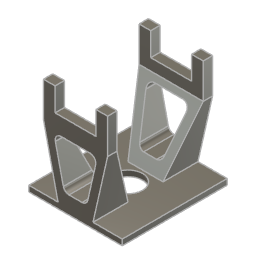
Jacks Stands F (Autodesk Fusion 360 design; units mm, degrees)
Autodesk Fusion 360 part; units mm, degrees
note: some values were not read from the file. Set by a fixed rule: which sketch regions a step uses.
sketch "Esquisse1" plane through (0, 0, 0) normal (0, 0, 1) x (1, 0, 0)
  line L0 (22.5, 70) -> (57.5, 70)
  line L1 (57.5, 70) -> (57.5, 90)
  line L2 (22.5, 70) -> (22.5, 90)
  line L3 (22.5, 90) -> (12.5, 90)
  line L4 (57.5, 90) -> (67.5, 90)
  line L5 (67.5, 90) -> (67.5, 60)
  line L6 (12.5, 90) -> (12.5, 60)
  line L7 (12.5, 60) -> (25, 5)
  line L8 (25, 5) -> (0, 5)
  line L9 (0, 5) -> (0, 0)
  line L10 (0, 0) -> (80, 0)
  line L11 (80, 0) -> (80, 5)
  line L12 (80, 5) -> (55, 5)
  line L13 (55, 5) -> (67.5, 60)
  dimension "d1" = 70
  dimension "d2" = 35
  dimension "d3" = 20
  dimension "d4" = 10
  dimension "d5" = 30
  dimension "d8" = 5
  dimension "d10" = 10
  dimension "d27" = 80
  dimension "d28" = 55
  dimension "d29" = 12.5
  dimension "d30" = 30
  constraint horizontal L0
  constraint perpendicular L0 L1
  constraint perpendicular L0 L2
  constraint perpendicular L2 L3
  constraint perpendicular L1 L4
  constraint perpendicular L4 L5
  constraint equal L3 L4
  constraint perpendicular L3 L6
  constraint perpendicular L6 L8
  constraint coincident L9.end L10.start
  constraint perpendicular L8 L9
  constraint perpendicular L9 L10
  constraint perpendicular L10 L11
  constraint perpendicular L9 L12
  constraint horizontal L5.end L6.end
  constraint equal L8 L12
  constraint collinear L8 L12
  measures "d1" distance of L9.end L0
  measures "d2" distance of L0.start L0.end
  measures "d3" distance of L0.end L1.end
  measures "d4" distance of L2.end L3.end
  measures "d5" distance of L3.end L6.end
  measures "d8" distance of L8 L10
  measures "d10" vertical distance of L0.end L5.end
  measures "d27" distance of L9.end L10.end
  measures "d28" distance of L5 L6
  measures "d29" distance of L5 L11
  measures "d30" distance of L7.end L12.end
extrude "Extrusion1" add sketch "Esquisse1" along normal blind 90
sketch "Esquisse2" plane through (67.5, 0, 0) normal (1, 0, 0) x (0, 0, -1)
  line L0 (0, 60) -> (0, 90)
  line L1 (0, 90) -> (-90, 90)
  line L2 (-90, 90) -> (-90, 60)
  line L3 (-90, 60) -> (0, 60)
  line L4 (-45, 90) -> (-45, -26) construction
  line L5 (-82, 90) -> (-82, 60)
  line L6 (-82, 60) -> (-60, 5)
  line L7 (-8, 90) -> (-8, 60)
  line L8 (-8, 60) -> (-30, 5)
  line L9 (-60, 5) -> (-30, 5)
  point P0 (-90, 5)
  point P1 (0, 5)
  dimension "d13" = 8
  dimension "d15" = 30
  dimension "d16" = 8
  dimension "d33" = 30
  constraint midpoint L1 L4.start
  constraint perpendicular L1 L4
  constraint coincident L1 L5.start
  constraint coincident L3 L5.end
  constraint perpendicular L3 L5
  constraint horizontal L6.end P0
  constraint coincident L1 L7.start
  constraint coincident L3 L7.end
  constraint perpendicular L3 L7
  constraint horizontal L6.end L8.end
  measures "d13" distance of L2 L5
  measures "d15" distance of L8.end P1
  measures "d16" distance of L0.end L7.start
  measures "d33" distance of L6.end P0
extrude "Extrusion2" cut sketch "Esquisse2" against normal blind 60 contours L3 L6 L8 L9 | L1 L3 L5 L7
sketch "Esquisse3" plane through (0, 0, 90) normal (0, 0, 1) x (1, 0, 0)
  line L0 (22.5, 70) -> (22.5, 90)
  line L1 (22.5, 90) -> (12.5, 90)
  line L2 (12.5, 90) -> (12.5, 60)
  line L3 (12.5, 60) -> (25, 5)
  line L4 (55, 5) -> (67.5, 60)
  line L5 (67.5, 60) -> (67.5, 90)
  line L6 (67.5, 90) -> (57.5, 90)
  line L7 (57.5, 90) -> (57.5, 70)
  line L8 (57.5, 70) -> (22.5, 70)
  line L9 (22.7158, 48.8919) -> (29.534, 18.8919)
  line L10 (34.4097, 15) -> (45.5903, 15)
  line L11 (50.466, 18.8919) -> (57.2842, 48.8919)
  line L12 (52.4085, 55) -> (27.5915, 55)
  arc A0 (27.5915, 55) -> (22.7158, 48.8919) centre (27.5915, 50) ccw
  arc A1 (57.2842, 48.8919) -> (52.4085, 55) centre (52.4085, 50) ccw
  arc A2 (29.534, 18.8919) -> (34.4097, 15) centre (34.4097, 20) ccw
  arc A3 (45.5903, 15) -> (50.466, 18.8919) centre (45.5903, 20) ccw
  line L13 (25, 5) -> (0, 5)
  line L14 (0, 5) -> (0, 0)
  line L15 (0, 0) -> (80, 0)
  line L16 (80, 0) -> (80, 5)
  line L17 (80, 5) -> (55, 5)
  dimension "d20" = 15
  dimension "d21" = 7.5
  dimension "d22" = 7.5
  dimension "d25" = 5
  constraint horizontal L10
  constraint parallel L10 L12
  constraint parallel L3 L9
  constraint parallel L4 L11
  constraint tangent L9 A0
  constraint tangent L12 A0
  constraint tangent L11 A1
  constraint tangent L12 A1
  constraint equal A0 A1
  constraint tangent L9 A2
  constraint tangent L10 A2
  constraint equal A0 A2
  constraint tangent L10 A3
  constraint tangent L11 A3
  constraint equal A0 A3
  measures "d20" distance of L8 L12
  measures "d21" distance of L4 L11
  measures "d22" distance of L3 L9
  measures "d25" radius of A0
extrude "Extrusion3" cut sketch "Esquisse3" against normal blind 150 contours L9 L10 L11 L12 A0 A1 A2 A3
sketch "Esquisse4" plane through (0, 5, 0) normal (0, 1, 0) x (-1, 0, 0)
  line L0 (-55, 90) -> (-80, 90)
  line L1 (-80, 90) -> (-80, 0)
  line L2 (-80, 0) -> (-55, 0)
  line L3 (-55, 30) -> (-25, 30)
  line L4 (-25, 30) -> (-25, 0)
  line L5 (-25, 0) -> (0, 0)
  line L6 (0, 0) -> (0, 90)
  line L7 (-55, 0) -> (-55, 30)
  line L8 (0, 90) -> (-25, 90)
  circle A0 centre (-40, 45) radius 12.5
  dimension "d34" = 25
  measures "d34" diameter of A0
extrude "Extrusion4" cut sketch "Esquisse4" against normal blind 20
equation "d14 = 30 mm"
equation "d15 = d14"
equation "d16 = d13"
equation "d29 = ( d27 - d28 ) / 2"
equation "d33 = d15"
